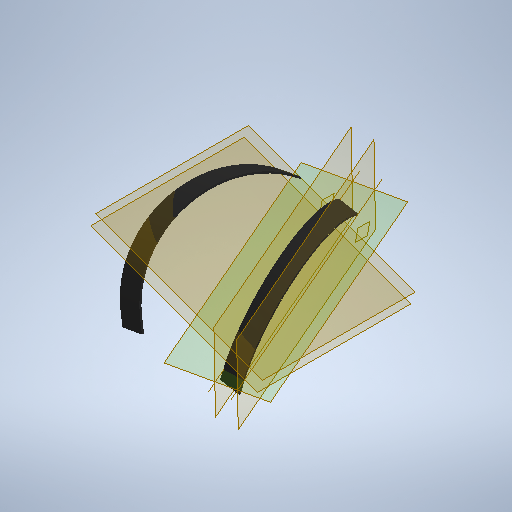
# Autodesk Inventor part: belt
Saved by Autodesk Inventor 2026.1 (Build 301233020, 233B)
## iProperties
Created: 2026-02-04
Part Number: belt
Material: 一般
Document SubType Name: Modeling
Designer: hibik
Density: 1 g/cm^3
Appearance: 既定
Author: hibik
Autodesk Inventor part; units mm, degrees
ref_plane "XY Plane" through (0, 0, 0) normal (0, 0, 1) x (1, 0, 0)
ref_plane "作業平面2" through (70.6693, 25.9112, 12.5) normal (0.9287275, -0.2499237, -0.2738674) x (0.1523203, -0.4162505, 0.8964006)
ref_plane "作業平面1" through (70.6693, 25.9112, 12.5) normal (0, -0.906984, -0.421165) x (0.1523203, -0.4162505, 0.8964006)
ref_plane "作業平面5" through (72.5487, 25.2272, 16.5) normal (0.9848078, -0.1736482, 0) x (0, 0, 1)
ref_plane "作業平面4" through (0, 0, 0) normal (0.9848078, -0.1736482, 0) x (0, 0, 1)
sketch "スケッチ4" plane through (72.5487, 25.2272, 16.5) normal (0.9848078, -0.1736482, 0) x (0, 0, 1)
  arc A0 (-4, -0.3473) -> (251, 108.7407) centre (93.9958, 123.1646) ccw
  arc A1 (-2.1354, 2.0028) -> (248.0126, 109.0151) centre (93.9958, 123.1646) ccw
  line L0 (-2.1354, 2.0028) -> (-4, -0.3473)
  line L1 (251, 108.7407) -> (248.0126, 109.0151)
  line L2 (251, 108.7407) -> (248.0126, 109.0151)
  line L3 (248.0126, 109.0151) -> (250.285, 133.7505)
  line L4 (250.285, 133.7505) -> (253.2724, 133.476)
  line L5 (253.2724, 133.476) -> (251, 108.7407)
  point P0 (-16.5, 37.4419)
  dimension "d10" = 3
  constraints: 12 end point, 4 point on circle, 3 equal length, 2 centre point, 1 perpendicular, 2 other
  measures "d10" radial gap between concentric circles of A0 A1
extrude "押し出し4" add sketch "スケッチ4" along normal mid plane 200
sketch "スケッチ5" plane through (70.6693, 25.9112, 12.5) normal (0.9287275, -0.2499237, -0.2738674) x (0.1523203, -0.4162505, 0.8964006)
  line L0 (-182.7887, -200.8557) -> (555.7515, -200.8557)
  line L1 (555.7515, -200.8557) -> (555.7515, 275.1143)
  line L2 (555.7515, 275.1143) -> (-182.7887, 275.1143)
  line L3 (-182.7887, 275.1143) -> (-182.7887, -200.8557)
  point P0 (-11.1838, 50.897)
  constraints: 8 end point, 2 parallel, 1 horizontal, 1 perpendicular
extrude "押し出し5" cut sketch "スケッチ5" along normal through all
ref_plane "作業平面6" through (38.1638, 34.6585, 22.0854) normal (0.9287275, -0.2499237, -0.2738674) x (0.1523203, -0.4162505, 0.8964006)
sketch "スケッチ6" plane through (38.1638, 34.6585, 22.0854) normal (0.9287275, -0.2499237, -0.2738674) x (0.1523203, -0.4162505, 0.8964006)
  line L0 (-129.6846, -185.1212) -> (393.489, -185.1212)
  line L1 (393.489, -185.1212) -> (393.489, 176.7734)
  line L2 (393.489, 176.7734) -> (-129.6846, 176.7734)
  line L3 (-129.6846, 176.7734) -> (-129.6846, -185.1212)
  point P0 (-11.1838, 50.897)
  constraints: 8 end point, 2 parallel, 1 horizontal, 1 perpendicular
extrude "押し出し6" cut sketch "スケッチ6" against normal through all
mirror "ミラー1" about plane through (0, 0, 0) normal (1, 0, 0)
ref_plane "作業平面8" through (141.4575, -77.8279, 12.5) normal (0.3420201, 0.9396926, 0) x (0, 0, 1)
ref_plane "作業平面7" through (0, 0, 0) normal (0.3420201, 0.9396926, 0) x (0, 0, 1)
